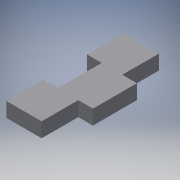
# Autodesk Inventor part: Part14
Saved by Autodesk Inventor 2019 (Build 230136000, 136)
## iProperties
Created: 2018-05-22
Part Number: Part14
Material: Generic
Document SubType Name: Modeling
Designer: Jerry
Density: 1 g/cm^3
Appearance: Default
Author: Jerry
Autodesk Inventor part; units mm, degrees
ref_plane "YZ Plane" through (0, 0, 0) normal (1, 0, 0) x (0, 1, 0)
ref_plane "XZ Plane" through (0, 0, 0) normal (0, 1, 0) x (-1, 0, 0)
ref_plane "XY Plane" through (0, 0, 0) normal (0, 0, 1) x (1, 0, 0)
sketch "Sketch1" plane through (0, 0, 0) normal (0, 1, 0) x (-1, 0, 0)
  line L0 (5.2556, 29.8923) -> (-2.3644, 29.8923)
  line L1 (-2.3644, 29.8923) -> (-2.3644, 4.4923)
  line L2 (-2.3644, 4.4923) -> (5.2556, 4.4923)
  line L3 (5.2556, 4.4923) -> (5.2556, 29.8923)
  line L4 (-2.3644, 21.9548) -> (-5.5394, 21.9548)
  line L5 (-5.5394, 21.9548) -> (-5.5394, 12.4298)
  line L6 (-5.5394, 12.4298) -> (-2.3644, 12.4298)
  line L7 (-2.3644, 12.4298) -> (-2.3644, 21.9548)
  line L8 (5.2556, 12.4298) -> (2.0806, 12.4298)
  line L9 (2.0806, 12.4298) -> (2.0806, 21.9548)
  line L10 (2.0806, 21.9548) -> (5.2556, 21.9548)
  line L11 (5.2556, 21.9548) -> (5.2556, 12.4298)
  point P0 (0, 0)
  dimension "d0" = 25.4
  dimension "d1" = 3.175
  dimension "d2" = 7.62
  dimension "d3" = 7.9375
  dimension "d4" = 7.9375
  dimension "d7" = 3.175
  constraints: 24 end point, 6 parallel, 3 horizontal, 3 perpendicular, 2 point on line
  measures "d0" distance between parallel lines of L2 L0
  measures "d1" distance between parallel lines of L1 L5
  measures "d2" distance between parallel lines of L3 L1
  measures "d3" distance between parallel lines of L2 L6
  measures "d4" distance between parallel lines of L4 L0
  measures "d7" distance between parallel lines of L9 L3
extrude "Extrusion2" add sketch "Sketch1" along normal blind 3.175 contours L3 L10 L9 L8 L2 L1 L0 | L1 L6 L5 L4
body "Solid2"
